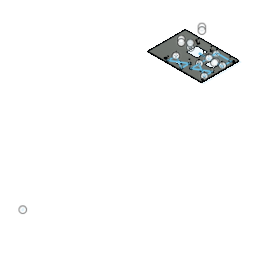
lid (Autodesk Fusion 360 design; units mm, degrees)
Autodesk Fusion 360 part; units mm, degrees
note: some values were not read from the file. Chosen so that the rebuilt part matches the saved one: which bodies a step acts on. Set by a fixed rule: which sketch regions a step uses; which face or edge a step refers to.
sketch "Sketch1" plane through (0, 0, 0) normal (0, 0, 1) x (1, 0, 0)
sketch "Sketch2" plane through (0, 0, 0) normal (1, 0, 0) x (0, 1, 0)
  line L0 (32, 8.9863) -> (32, 4)
  line L1 (-0.5157, 4) -> (-0.5157, 8.9863)
  circle A0 centre (-249.9, -99.15) radius 0.8
  constraint vertical L0
  constraint vertical L1
sketch "Sketch3" plane through (0, 0, 0) normal (0, 0, 1) x (1, 0, 0)
  circle A0 centre (4, 3.7) radius 0.8
extrude "Extrude1" add sketch "Sketch3" along normal blind 5 makes body 1
extrude "Extrude2" add 1 faces at (3.8681, 4.0199, 5) along direction (0, 0, 1) blind 1.5 on bodies 1 bodies 1
move_body "Move1" bodies 1 to x (1, 0, 0) y (0, 1, 0) z (0, 0, 1) at (0, 10, 0)
copy_body "CopyPasteBodies1" bodies 1 makes body 2
copy_body "CopyPasteBodies2" bodies 2 makes body 3
move_body "Move2" bodies 3 to x (1, 0, 0) y (0, 1, 0) z (0, 0, 1) at (0, -10, 0)
move_body "Move3" bodies 2 to x (1, 0, 0) y (0, 1, 0) z (0, 0, 1) at (0, 2.7, 0)
copy_body "CopyPasteBodies3" bodies 3 makes body 4
move_body "Move4" bodies 4 to x (1, 0, 0) y (0, 1, 0) z (0, 0, 1) at (21, 0, 0)
move_body "Move5" bodies 1 to x (1, 0, 0) y (0, 1, 0) z (0, 0, 1) at (21, 2.7, 0)
copy_body "CopyPasteBodies4" bodies 1 2 3 4 makes body 5 makes body 6 makes body 7 makes body 8
move_body "Move6" bodies 5 6 7 8 to x (1, 0, 0) y (0, 1, 0) z (0, 0, 1) at (26, 0, 0)
sketch "Sketch4" plane through (0, 0, 0) normal (0, 0, 1) x (1, 0, 0)
  line L0 (-9.0529, 25.1435) -> (80, 25.1435)
  line L1 (80, 25.1435) -> (80, -35)
  line L2 (80, -35) -> (-9.0529, -35)
  line L3 (-9.0529, -35) -> (-9.0529, 25.1435)
  constraint horizontal L0
  constraint vertical L1
  constraint horizontal L2
  constraint vertical L3
move_body "Move7" bodies 5 6 7 8 to x (1, 0, 0) y (0, 1, 0) z (0, 0, 1) at (1, 0, 0)
sketch "Sketch5" plane through (0, 0, 0) normal (0, 0, 1) x (1, 0, 0)
  line L0 (38.2, 17.2) -> (60.7999, 17.2)
  line L1 (60.7999, 17.2) -> (60.7999, 2.9046)
  line L2 (60.7999, 2.9046) -> (38.2, 2.9046)
  line L3 (38.2, 2.9046) -> (38.2, 17.2)
  line L4 (60.7999, 2.9046) -> (25.8, 2.9046)
  line L5 (25.8, 2.9046) -> (25.8, 2.9)
  line L6 (25.8, 2.9) -> (60.7999, 2.9)
  line L7 (60.7999, 2.9) -> (60.7999, 2.9046)
  constraint horizontal L0
  constraint vertical L1
  constraint horizontal L2
  constraint vertical L3
  constraint horizontal L4
  constraint vertical L5
  constraint horizontal L6
  constraint vertical L7
move_body "Move8" bodies 1 4 8 6 2 5 7 3 to x (1, 0, 0) y (0, 1, 0) z (0, 0, 1) at (10, 0, 0)
copy_body "CopyPasteBodies5" bodies 5 6 7 8 makes body 9 makes body 10 makes body 11 makes body 12
move_body "Move9" bodies 9 10 11 12 to x (1, 0, 0) y (0, 1, 0) z (0, 0, 1) at (0, -27, 0)
copy_body "CopyPasteBodies6" bodies 9 10 11 12 makes body 13 makes body 14 makes body 15 makes body 16
move_body "Move10" bodies 13 14 15 16 to x (1, 0, 0) y (0, 1, 0) z (0, 0, 1) at (-27, 0, 0)
move_body "Move11" bodies 3 15 1 4 14 2 13 16 to x (1, 0, 0) y (0, 1, 0) z (0, 0, 1) at (-2, 0, 0)
sketch "Sketch6" plane through (0, 0, 0) normal (0, 0, 1) x (1, 0, 0)
move_body "Move12" bodies 14 11 4 7 3 2 8 5 13 12 9 6 1 16 15 10 to x (1, 0, 0) y (0, 1, 0) z (0, 0, 1) at (-2, 0, 0)
extrude "Extrude3" add sketch "Sketch4" against normal blind 1 bodies 1 2 3 4 5 6 7 8 9 10 11 12 13 14 15 16
sketch "Sketch7" plane through (0, 0, 0) normal (0, 0, 1) x (-1, 0, 0)
  circle A0 centre (-10, 23.3) radius 0.8
  circle A1 centre (-31, 10.6) radius 0.8
  circle A2 centre (-39, 23.3) radius 0.8
  circle A3 centre (-60, 10.6) radius 0.8
  circle A4 centre (-39, -3.7) radius 0.8
  circle A5 centre (-60, -16.4) radius 0.8
  circle A6 centre (-10, -3.7) radius 0.8
  circle A7 centre (-31, -16.4) radius 0.8
  circle A8 centre (-10, -16.4) radius 0.8
  circle A9 centre (-31, -3.7) radius 0.8
  circle A10 centre (-39, -16.4) radius 0.8
  circle A11 centre (-60, -3.7) radius 0.8
  circle A12 centre (-39, 10.6) radius 0.8
  circle A13 centre (-60, 23.3) radius 0.8
  circle A14 centre (-10, 10.6) radius 0.8
  circle A15 centre (-31, 23.3) radius 0.8
  line L0 (9.0529, 35) -> (-80, 35)
  line L1 (-80, 35) -> (-80, -25.1435)
  line L2 (-80, -25.1435) -> (9.0529, -25.1435)
  line L3 (9.0529, -25.1435) -> (9.0529, 35)
  line L4 (-10, -16.4) -> (-28.4563, -16.4)
  line L5 (-28.4563, -16.4) -> (-28.4563, -3.2)
  line L6 (-28.4563, -3.2) -> (-10, -3.2)
  line L7 (-10, -3.2) -> (-10, -16.4)
  constraint horizontal L4
  constraint vertical L5
  constraint horizontal L6
  constraint vertical L7
  constraint coincident A8.centre L4.start
sketch "Sketch8" plane through (0, 0, 0) normal (0, 0, 1) x (1, 0, 0)
  line L0 (49.5, 4.5) -> (49.5, 2.2044)
  constraint vertical L0
sketch "Sketch9" plane through (0, 0, 0) normal (0, 0, 1) x (1, 0, 0)
  line L0 (12.5, -2) -> (28.5, -2)
  line L1 (28.5, -2) -> (28.5, 14)
  line L2 (28.5, 14) -> (12.5, 14)
  line L3 (12.5, 14) -> (12.5, -2)
  line L4 (28.5, 14) -> (12.5, 14)
  line L5 (12.5, 14) -> (12.5, -2)
  line L6 (12.5, -2) -> (28.5, -2)
  line L7 (28.5, -2) -> (28.5, 14)
  line L8 (12.5, -2) -> (28.5, -2)
  line L9 (28.5, -2) -> (28.5, 14)
  line L10 (28.5, 14) -> (12.5, 14)
  line L11 (12.5, 14) -> (12.5, -2)
  line L12 (12.5, 14) -> (28.5, 14)
  line L13 (28.5, 14) -> (28.5, -2)
  line L14 (28.5, -2) -> (12.5, -2)
  line L15 (12.5, -2) -> (12.5, 14)
  constraint horizontal L0
  constraint vertical L1
  constraint horizontal L2
  constraint vertical L3
  constraint horizontal L4
  constraint vertical L5
  constraint horizontal L6
  constraint vertical L7
  constraint horizontal L8
  constraint vertical L9
  constraint horizontal L10
  constraint vertical L11
  constraint horizontal L12
  constraint vertical L13
  constraint horizontal L14
  constraint vertical L15
extrude "Extrude4" cut sketch "Sketch9" along normal blind 1 and the other way blind 7 bodies 1
sketch "Sketch10" plane through (0, 0, 0) normal (0, 0, 1) x (-1, 0, 0)
  line L0 (-39, -15.6) -> (-39, -4.5)
  constraint vertical L0
sketch "Sketch11" plane through (0, 0, 0) normal (0, 0, 1) x (-1, 0, 0)
  line L0 (-39, -4.5) -> (-60, -4.5)
  constraint horizontal L0
sketch "Sketch12" plane through (0, 0, 0) normal (0, 0, 1) x (1, 0, 0)
  line L0 (43.75, 4.5) -> (55.25, 4.5)
  line L1 (55.25, 4.5) -> (55.25, -7)
  line L2 (55.25, -7) -> (43.75, -7)
  line L3 (43.75, -7) -> (43.75, 4.5)
  constraint horizontal L0
  constraint vertical L1
  constraint horizontal L2
  constraint vertical L3
extrude "Extrude5" cut sketch "Sketch12" along normal blind 2 and the other way blind 4 bodies 1
sketch "Sketch13" plane through (0, 0, 0) normal (0, 0, 1) x (1, 0, 0)
  line L0 (39, 2.9) -> (39, -11)
  constraint vertical L0
move_face "MoveFace1" to x (1, 0, 0) y (0, 1, 0) z (0, 0, 1) at (0, 0, 6) 1 faces at (30.3174, 15.9829, 4.3333) on bodies 1
split "Split1" by plane through (0, 0, 0) normal (0, 0, 1) bodies 1 makes body 17 at (9.201, -23.3399, 4.3333) makes body 18 at (10.796, -10.6797, 4.3333) makes body 19 at (31.796, -10.6797, 4.3333) makes body 20 at (60.365, -22.5881, 2.1667) makes body 21 at (39.365, -22.5881, 2.1667) makes body 22 at (39.1389, -9.8122, 2.1667) makes body 23 at (60.1389, -9.8122, 2.1667) makes body 24 at (60.1389, 4.4878, 2.1667) makes body 25 at (39.1389, 4.4878, 2.1667) makes body 26 at (39.0995, 15.6062, 2.1667) makes body 27 at (60.0995, 15.6062, 2.1667) makes body 28 at (31.796, 3.6203, 4.3333) makes body 29 at (10.796, 3.6203, 4.3333) makes body 30 at (9.201, 16.3601, 4.3333) makes body 31 at (30.3174, 15.9829, 4.3333) makes body 32 at (30.201, -23.3399, 4.3333)
move_face "MoveFace2" to x (1, 0, 0) y (0, 1, 0) z (0, 0, 1) at (0, -7, 0) 4 faces at (9.201, -23.3399, 4.3333) (10.796, -10.6797, 4.3333) (31.796, -10.6797, 4.3333) (30.201, -23.3399, 4.3333) on bodies 17 18 19 32
move_face "MoveFace3" to x (1, 0, 0) y (0, 1, 0) z (0, 0, 1) at (0, -1, 0) 8 faces at (39.1389, -9.8122, 2.1667) (60.1389, -9.8122, 2.1667) (60.365, -22.5881, 2.1667) (39.365, -22.5881, 2.1667) (30.201, -17.6399, 4.3333) (9.201, -17.6399, 4.3333) (9.201, -30.3399, 4.3333) (30.201, -30.3399, 4.3333) on bodies 17 18 19 20 21 22 23 32
sketch "Sketch14" plane through (0, 0, 0) normal (0, 0, 1) x (-1, 0, 0)
  line L0 (-10, 19.4) -> (-10, 31.3)
  line L1 (-10, 31.3) -> (-31, 18.6)
  line L2 (-31, 18.6) -> (-31, 31.3)
  line L3 (-31, 31.3) -> (-10, 18.6)
  constraint vertical L0
  constraint parallel L0 L2
hole "Hole1" at (20.5009, -24.9504, 0) direction (0, 0, -1) diameter 5.55 depth 5 tip angle 118 bodies 1
sketch "Sketch15" plane through (0, 0, 0) normal (0, 0, 1) x (-1, 0, 0)
  line L0 (-39, 11.6) -> (-39, 24.3)
  line L1 (-39, 24.3) -> (-60, 11.6)
  line L2 (-60, 11.6) -> (-60, 24.3)
  line L3 (-60, 24.3) -> (-39, 11.6)
  constraint vertical L0
  constraint parallel L0 L2
sketch "Sketch16" plane through (0, 0, 0) normal (0, 0, 1) x (-1, 0, 0)
  line L0 (-50.4991, 15.8331) -> (-48.5009, 15.8331)
  line L1 (-48.5009, 15.8331) -> (-48.5009, 20.0669)
  line L2 (-48.5009, 20.0669) -> (-50.4991, 20.0669)
  line L3 (-50.4991, 20.0669) -> (-50.4991, 15.8331)
  line L4 (-50.4991, 15.8331) -> (-48.5009, 20.0669) construction
  line L5 (-48.5009, 15.8331) -> (-50.4991, 20.0669) construction
  point P0 (-49.5, 17.95)
  constraint horizontal L0
  constraint perpendicular L0 L1
  constraint parallel L0 L2
  constraint parallel L1 L3
  constraint coincident L4 P0
  constraint coincident L5 P0
extrude "Extrude6" cut sketch "Sketch16" along normal blind 1.5 and the other way blind 1.5 bodies 1
sketch "Sketch17" plane through (0, 0, 0) normal (1, 0, 0) x (0, 1, 0)
  line L0 (3.7, 0, 10) -> (3.7, 6.5, 10)
chamfer "Chamfer2" distance 0.25 angle 45 16 edges at (38.2541, -11.8893, 6.5) (9.2541, -18.8893, 6.5) (59.2541, 3.4107, 6.5) (9.2541, -31.5893, 6.5) (59.2541, -11.8893, 6.5) (30.2541, -18.8893, 6.5) (30.2541, 16.1107, 6.5) (30.2541, -31.5893, 6.5) (38.2541, 3.4107, 6.5) (38.2541, 16.1107, 6.5) (9.2541, 3.4107, 6.5) (9.2541, 16.1107, 6.5) (59.2541, -24.5893, 6.5) (59.2541, 16.1107, 6.5) (30.2541, 3.4107, 6.5) (38.2541, -24.5893, 6.5) on bodies 2 3 4 5 6 7 8 17 18 19 20 21 22 23 24 25 26 27 28 29 30 31 32
fillet "Fillet1" radius 0.1 4 edges at (43.75, -7, -0.5) (43.75, 4.5, -0.5) (55.25, -7, -0.5) (55.25, 4.5, -0.5) on bodies 1
fillet "Fillet2" radius 0.1 4 edges at (48.5009, -15.8331, -0.5) (50.4991, -15.8331, -0.5) (48.5009, -20.0669, -0.5) (50.4991, -20.0669, -0.5) on bodies 1
fillet "Fillet3" radius 0.1 4 edges at (28.5, -2, -0.5) (28.5, 14, -0.5) (12.5, 14, -0.5) (12.5, -2, -0.5) on bodies 1
fillet "Fillet6" radius 0.075 1 edges at (17.9137, -23.9469, 0) on bodies 1
sketch "Sketch18" plane through (0, 0, 0) normal (0, 0, 1) x (-1, 0, 0)
  circle A0 centre (-60, 24.3) radius 1.2728
sketch "Sketch19" plane through (0, 0, 0) normal (0, 0, 1) x (1, 0, 0)
  circle A0 centre (10, 16.4) radius 1.8028
extrude "Extrude7" add sketch "Sketch19" along normal blind 1.5 separate body makes body 33
sketch "Sketch20" plane through (0, 0, 0) normal (0, 0, 1) x (-1, 0, 0)
  circle A0 centre (-31, -16.4) radius 1.75
  dimension "d38" = 3.5
  measures "d38" diameter of A0
extrude "Extrude8" add sketch "Sketch20" along normal blind 1.5 separate body makes body 34
sketch "Sketch21" plane through (0, 0, 0) normal (0, 0, 1) x (-1, 0, 0)
  circle A0 centre (-39, -16.4) radius 1.75
  dimension "d41" = 3.5
  measures "d41" diameter of A0
extrude "Extrude9" add sketch "Sketch21" along normal blind 1.5 separate body makes body 35
sketch "Sketch22" plane through (0, 0, 0) normal (0, 0, 1) x (-1, 0, 0)
  circle A0 centre (-39, -3.7) radius 1.75
  dimension "d44" = 3.5
  measures "d44" diameter of A0
extrude "Extrude10" add sketch "Sketch22" along normal blind 1.5 separate body makes body 36
sketch "Sketch23" plane through (0, 0, 0) normal (0, 0, 1) x (-1, 0, 0)
  circle A0 centre (-31, -3.7) radius 1.75
  dimension "d47" = 3.5
  measures "d47" diameter of A0
extrude "Extrude11" add sketch "Sketch23" along normal blind 1.5 separate body makes body 37
sketch "Sketch24" plane through (0, 0, 0) normal (0, 0, 1) x (-1, 0, 0)
  circle A0 centre (-39, 11.6) radius 1.75
  dimension "d50" = 3.5
  measures "d50" diameter of A0
extrude "Extrude12" add sketch "Sketch24" along normal blind 1.5 separate body makes body 38
sketch "Sketch25" plane through (0, 0, 0) normal (0, 0, 1) x (-1, 0, 0)
  circle A0 centre (-60, -16.4) radius 1.75
  dimension "d53" = 3.5
  measures "d53" diameter of A0
extrude "Extrude13" add sketch "Sketch25" along normal blind 1.5 separate body makes body 39
sketch "Sketch26" plane through (0, 0, 0) normal (0, 0, 1) x (-1, 0, 0)
  circle A0 centre (-60, -3.7) radius 1.75
  dimension "d56" = 3.5
  measures "d56" diameter of A0
extrude "Extrude14" add sketch "Sketch26" along normal blind 1.5 separate body makes body 40
sketch "Sketch27" plane through (0, 0, 0) normal (0, 0, 1) x (-1, 0, 0)
  circle A0 centre (-60, 11.6) radius 1.75
  dimension "d59" = 3.5
  measures "d59" diameter of A0
extrude "Extrude15" add sketch "Sketch27" along normal blind 1.5 separate body makes body 41
sketch "Sketch28" plane through (0, 0, 0) normal (0, 0, 1) x (-1, 0, 0)
  circle A0 centre (-60, 24.3) radius 1.75
  dimension "d62" = 3.5
  measures "d62" diameter of A0
extrude "Extrude16" add sketch "Sketch28" along normal blind 1.5 separate body makes body 42
sketch "Sketch29" plane through (0, 0, 0) normal (0, 0, 1) x (-1, 0, 0)
  circle A0 centre (-39, 24.3) radius 1.75
  dimension "d65" = 3.5
  measures "d65" diameter of A0
extrude "Extrude17" add sketch "Sketch29" along normal blind 1.5 separate body makes body 43
sketch "Sketch30" plane through (0, 0, 0) normal (0, 0, 1) x (-1, 0, 0)
  circle A0 centre (-31, 18.6) radius 1.7499
extrude "Extrude18" cut sketch "Sketch30" along normal blind 1.5 bodies 19
sketch "Sketch31" plane through (0, 0, 0) normal (0, 0, 1) x (-1, 0, 0)
  circle A0 centre (-10, -3.7) radius 1.75
  dimension "d70" = 3.5
  measures "d70" diameter of A0
extrude "Extrude19" add sketch "Sketch31" along normal blind 1.5 separate body makes body 44
sketch "Sketch32" plane through (0, 0, 0) normal (0, 0, 1) x (-1, 0, 0)
  circle A0 centre (-10, 18.6) radius 1.75
  dimension "d73" = 3.5
  measures "d73" diameter of A0
extrude "Extrude20" add sketch "Sketch32" along normal blind 1.5 separate body makes body 45
sketch "Sketch33" plane through (0, 0, 0) normal (0, 0, 1) x (-1, 0, 0)
  circle A0 centre (-31, 18.6) radius 1.75
  dimension "d76" = 3.5
  measures "d76" diameter of A0
extrude "Extrude21" add sketch "Sketch33" along normal blind 1.5 bodies 1 19
sketch "Sketch34" plane through (0, 0, 0) normal (0, 0, 1) x (-1, 0, 0)
  circle A0 centre (-31, 31.3) radius 1.75
  dimension "d79" = 3.5
  measures "d79" diameter of A0
extrude "Extrude22" add sketch "Sketch34" along normal blind 1.5 separate body makes body 46
sketch "Sketch35" plane through (0, 0, 0) normal (0, 0, 1) x (-1, 0, 0)
  circle A0 centre (-10, 31.3) radius 1.75
  dimension "d82" = 3.5
  measures "d82" diameter of A0
extrude "Extrude23" add sketch "Sketch35" along normal blind 1.5 separate body makes body 47
fillet "Fillet7" radius 0.5 4 edges at (-9.0529, 25.1435, -0.5) (80, 25.1435, -0.5) (80, -35, -0.5) (-9.0529, -35, -0.5) on bodies 1
sketch "Sketch36" plane through (0, 0, 0) normal (0, 0, 1) x (-1, 0, 0)
  line L0 (-1.7, 34.5) -> (-79.5, 34.5)
  line L1 (-79.5, 34.5) -> (-79.5, -24.7)
  line L2 (-79.5, -24.7) -> (-1.7, -24.7)
  line L3 (-1.7, -24.7) -> (-1.7, 34.5)
  constraint horizontal L0
  constraint vertical L1
  constraint horizontal L2
  constraint vertical L3
extrude "Extrude24" cut sketch "Sketch36" against normal blind 0.5 bodies 1 makes body 48 at (31.796, -18.5203, 3.0833)
move_body "Move13" bodies 45 18 47 17 44 29 30 33 34 31 26 35 39 27 24 40 25 36 28 37 48 38 22 43 21 23 41 20 42 32 46 to x (1, 0, 0) y (0, 1, 0) z (0, 0, 1) at (0, 0, -0.5)
move_face "MoveFace4" by (10.2, 0, 0) 1 faces at (-9.0529, -14.7855, -0.3333) on bodies 1
move_face "MoveFace5" by (10.2, 0, 0) 1 faces at (80, 4.929, -0.3333) on bodies 1
move_face "MoveFace6" by (10.2, 0, 0) 1 faces at (79.5, 4.9667, -0.3333) on bodies 1
move_face "MoveFace7" by (-20.4, 0, 0) 2 faces at (89.7, 4.9667, -0.3333) (90.2, 4.929, -0.3333) on bodies 1
move_face "MoveFace8" by (-20.4, 0, 0) 2 faces at (1.7, -14.7667, -0.3333) (1.1471, -14.7855, -0.3333) on bodies 1
sketch "Sketch37" plane through (0, 0, -0.5) normal (0, 0, 1) x (-1, 0, 0)
  circle A0 centre (-20.5009, 24.9504) radius 2.775
  arc A1 (-12.6, -14) -> (-12.5, -13.9) centre (-12.6, -13.9) ccw
  line L0 (-12.6, -14) -> (-28.4, -14)
  arc A2 (-28.5, -13.9) -> (-28.4, -14) centre (-28.4, -13.9) ccw
  line L1 (-28.5, -13.9) -> (-28.5, 1.9)
  arc A3 (-28.4, 2) -> (-28.5, 1.9) centre (-28.4, 1.9) ccw
  line L2 (-28.4, 2) -> (-12.6, 2)
  arc A4 (-12.5, 1.9) -> (-12.6, 2) centre (-12.6, 1.9) ccw
  line L3 (-12.5, 1.9) -> (-12.5, -13.9)
  arc A5 (-48.5009, 19.9669) -> (-48.6009, 20.0669) centre (-48.6009, 19.9669) ccw
  line L4 (-48.5009, 19.9669) -> (-48.5009, 15.9331)
  arc A6 (-48.6009, 15.8331) -> (-48.5009, 15.9331) centre (-48.6009, 15.9331) ccw
  line L5 (-48.6009, 15.8331) -> (-50.3991, 15.8331)
  arc A7 (-50.4991, 15.9331) -> (-50.3991, 15.8331) centre (-50.3991, 15.9331) ccw
  line L6 (-50.4991, 15.9331) -> (-50.4991, 19.9669)
  arc A8 (-50.3991, 20.0669) -> (-50.4991, 19.9669) centre (-50.3991, 19.9669) ccw
  line L7 (-50.3991, 20.0669) -> (-48.6009, 20.0669)
  arc A9 (-43.85, -4.5) -> (-43.75, -4.4) centre (-43.85, -4.4) ccw
  line L8 (-43.85, -4.5) -> (-55.15, -4.5)
  arc A10 (-55.25, -4.4) -> (-55.15, -4.5) centre (-55.15, -4.4) ccw
  line L9 (-55.25, -4.4) -> (-55.25, 6.9)
  arc A11 (-55.15, 7) -> (-55.25, 6.9) centre (-55.15, 6.9) ccw
  line L10 (-55.15, 7) -> (-43.85, 7)
  arc A12 (-43.75, 6.9) -> (-43.85, 7) centre (-43.85, 6.9) ccw
  line L11 (-43.75, 6.9) -> (-43.75, -4.4)
  line L12 (18.7, -24.7) -> (18.7, 34.5)
  line L13 (18.7, 34.5) -> (-69.3, 34.5)
  line L14 (-69.3, 34.5) -> (-69.3, -24.7)
  line L15 (-69.3, -24.7) -> (18.7, -24.7)
  line L16 (-8.2, -18.2) -> (-32.7552, -18.2)
  line L17 (-32.7552, -18.2) -> (-32.7552, -1.944)
  line L18 (-32.7552, -1.944) -> (-8.2, -1.944)
  line L19 (-8.2, -1.944) -> (-8.2, -18.2)
  line L20 (-10, -16.4) -> (-31, -16.4)
  line L21 (-10, -3.7) -> (-31, -3.7)
  constraint horizontal L16
  constraint vertical L17
  constraint horizontal L18
  constraint vertical L19
  constraint parallel L0 L20
  constraint perpendicular L1 L21
move_face "OffsetFaces1" offset 2.3 1 faces at (17.8667, 14, -0.6667) on bodies 1
move_face "OffsetFaces2" offset -2.3 1 faces at (17.8667, -2, -0.8333) on bodies 1
sketch "Sketch38" plane through (0, 0, -0.5) normal (0, 0, 1) x (-1, 0, 0)
  line L0 (-12.5, 4.2) -> (-12.5, -11.6)
  arc A0 (-12.6, -11.7) -> (-12.5, -11.6) centre (-12.6, -11.6) ccw
  line L1 (-12.6, -11.7) -> (-28.4, -11.7)
  arc A1 (-28.5, -11.6) -> (-28.4, -11.7) centre (-28.4, -11.6) ccw
  line L2 (-28.5, -11.6) -> (-28.5, 4.2)
  arc A2 (-28.4, 4.3) -> (-28.5, 4.2) centre (-28.4, 4.2) ccw
  line L3 (-28.4, 4.3) -> (-12.6, 4.3)
  arc A3 (-12.5, 4.2) -> (-12.6, 4.3) centre (-12.6, 4.2) ccw
  circle A4 centre (-20.5009, 24.9504) radius 2.775
  arc A5 (-48.5009, 19.9669) -> (-48.6009, 20.0669) centre (-48.6009, 19.9669) ccw
  line L4 (-48.5009, 19.9669) -> (-48.5009, 15.9331)
  arc A6 (-48.6009, 15.8331) -> (-48.5009, 15.9331) centre (-48.6009, 15.9331) ccw
  line L5 (-48.6009, 15.8331) -> (-50.3991, 15.8331)
  arc A7 (-50.4991, 15.9331) -> (-50.3991, 15.8331) centre (-50.3991, 15.9331) ccw
  line L6 (-50.4991, 15.9331) -> (-50.4991, 19.9669)
  arc A8 (-50.3991, 20.0669) -> (-50.4991, 19.9669) centre (-50.3991, 19.9669) ccw
  line L7 (-50.3991, 20.0669) -> (-48.6009, 20.0669)
  arc A9 (-43.85, -4.5) -> (-43.75, -4.4) centre (-43.85, -4.4) ccw
  line L8 (-43.85, -4.5) -> (-55.15, -4.5)
  arc A10 (-55.25, -4.4) -> (-55.15, -4.5) centre (-55.15, -4.4) ccw
  line L9 (-55.25, -4.4) -> (-55.25, 6.9)
  arc A11 (-55.15, 7) -> (-55.25, 6.9) centre (-55.15, 6.9) ccw
  line L10 (-55.15, 7) -> (-43.85, 7)
  arc A12 (-43.75, 6.9) -> (-43.85, 7) centre (-43.85, 6.9) ccw
  line L11 (-43.75, 6.9) -> (-43.75, -4.4)
  line L12 (18.7, -24.7) -> (18.7, 34.5)
  line L13 (18.7, 34.5) -> (-69.3, 34.5)
  line L14 (-69.3, 34.5) -> (-69.3, -24.7)
  line L15 (-69.3, -24.7) -> (18.7, -24.7)
  line L16 (18.7, -24.7) -> (15.2004, -24.7)
  line L17 (15.2004, -24.7) -> (15.2004, 34.5)
  line L18 (15.2004, 34.5) -> (18.7, 34.5)
  line L19 (18.7, 34.5) -> (18.7, -24.7)
  line L20 (18.7, 34.5) -> (-65.7727, 34.5)
  line L21 (-65.7727, 34.5) -> (-65.7727, 31)
  line L22 (-65.7727, 31) -> (18.7, 31)
  line L23 (18.7, 31) -> (18.7, 34.5)
  line L24 (18.7, -24.7) -> (-69.2998, -24.7)
  line L25 (-69.2998, -24.7) -> (-69.2998, -21.2)
  line L26 (-69.2998, -21.2) -> (18.7, -21.2)
  line L27 (18.7, -21.2) -> (18.7, -24.7)
  line L28 (-69.3, -24.7) -> (-65.8, -24.7)
  line L29 (-65.8, -24.7) -> (-65.8, -21.2)
  line L30 (-65.8, -21.2) -> (-69.3, -21.2)
  line L31 (-69.3, -21.2) -> (-69.3, -24.7)
  line L32 (-69.3, 34.5) -> (-65.8, 34.5)
  line L33 (-65.8, 34.5) -> (-65.8, 31)
  line L34 (-65.8, 31) -> (-69.3, 31)
  line L35 (-69.3, 31) -> (-69.3, 34.5)
  circle A13 centre (-65.7727, 31) radius 1.55
  dimension "d91" = 3.5
  dimension "d92" = 3.5
  dimension "d93" = 3.5
  dimension "d94" = 3.1
  constraint horizontal L16
  constraint vertical L17
  constraint horizontal L18
  constraint vertical L19
  constraint coincident L13 L17.end
  constraint coincident L12.start L15.end
  constraint horizontal L20
  constraint vertical L21
  constraint horizontal L22
  constraint vertical L23
  constraint coincident L12.end L13.start
  constraint horizontal L24
  constraint vertical L25
  constraint horizontal L26
  constraint vertical L27
  constraint horizontal L28
  constraint vertical L29
  constraint horizontal L30
  constraint vertical L31
  constraint coincident L14.end L15.start
  constraint horizontal L32
  constraint vertical L33
  constraint horizontal L34
  constraint vertical L35
  constraint coincident L13.end L14.start
  constraint coincident L21.end L22.start
  measures "d91" distance of L12.end L22.end
  measures "d92" distance of L12.start L26.end
  measures "d93" distance of L14.end L28.end
  measures "d94" diameter of A13
sketch "Sketch39" plane through (0, 0, -0.5) normal (0, 0, 1) x (-1, 0, 0)
  line L0 (-12.5, 4.2) -> (-12.5, -11.6)
  arc A0 (-12.6, -11.7) -> (-12.5, -11.6) centre (-12.6, -11.6) ccw
  line L1 (-12.6, -11.7) -> (-28.4, -11.7)
  arc A1 (-28.5, -11.6) -> (-28.4, -11.7) centre (-28.4, -11.6) ccw
  line L2 (-28.5, -11.6) -> (-28.5, 4.2)
  arc A2 (-28.4, 4.3) -> (-28.5, 4.2) centre (-28.4, 4.2) ccw
  line L3 (-28.4, 4.3) -> (-12.6, 4.3)
  arc A3 (-12.5, 4.2) -> (-12.6, 4.3) centre (-12.6, 4.2) ccw
  circle A4 centre (-20.5009, 24.9504) radius 2.775
  arc A5 (-48.5009, 19.9669) -> (-48.6009, 20.0669) centre (-48.6009, 19.9669) ccw
  line L4 (-48.5009, 19.9669) -> (-48.5009, 15.9331)
  arc A6 (-48.6009, 15.8331) -> (-48.5009, 15.9331) centre (-48.6009, 15.9331) ccw
  line L5 (-48.6009, 15.8331) -> (-50.3991, 15.8331)
  arc A7 (-50.4991, 15.9331) -> (-50.3991, 15.8331) centre (-50.3991, 15.9331) ccw
  line L6 (-50.4991, 15.9331) -> (-50.4991, 19.9669)
  arc A8 (-50.3991, 20.0669) -> (-50.4991, 19.9669) centre (-50.3991, 19.9669) ccw
  line L7 (-50.3991, 20.0669) -> (-48.6009, 20.0669)
  arc A9 (-43.85, -4.5) -> (-43.75, -4.4) centre (-43.85, -4.4) ccw
  line L8 (-43.85, -4.5) -> (-55.15, -4.5)
  arc A10 (-55.25, -4.4) -> (-55.15, -4.5) centre (-55.15, -4.4) ccw
  line L9 (-55.25, -4.4) -> (-55.25, 6.9)
  arc A11 (-55.15, 7) -> (-55.25, 6.9) centre (-55.15, 6.9) ccw
  line L10 (-55.15, 7) -> (-43.85, 7)
  arc A12 (-43.75, 6.9) -> (-43.85, 7) centre (-43.85, 6.9) ccw
  line L11 (-43.75, 6.9) -> (-43.75, -4.4)
  line L12 (18.7, -24.7) -> (18.7, 34.5)
  line L13 (18.7, 34.5) -> (-69.3, 34.5)
  line L14 (-69.3, 34.5) -> (-69.3, -24.7)
  line L15 (-69.3, -24.7) -> (18.7, -24.7)
  line L16 (-69.3, -24.7) -> (-65.8, -24.7)
  line L17 (-65.8, -24.7) -> (-65.8, -21.2)
  line L18 (-65.8, -21.2) -> (-69.3, -21.2)
  line L19 (-69.3, -21.2) -> (-69.3, -24.7)
  circle A13 centre (-65.8, -21.2) radius 1.55
  dimension "d97" = 3.1
  constraint horizontal L16
  constraint vertical L17
  constraint horizontal L18
  constraint vertical L19
  constraint coincident L14.end L15.start
  constraint coincident L17.end L18.start
  measures "d97" diameter of A13
sketch "Sketch40" plane through (0, 0, -0.5) normal (0, 0, 1) x (-1, 0, 0)
  line L0 (-12.5, 4.2) -> (-12.5, -11.6)
  arc A0 (-12.6, -11.7) -> (-12.5, -11.6) centre (-12.6, -11.6) ccw
  line L1 (-12.6, -11.7) -> (-28.4, -11.7)
  arc A1 (-28.5, -11.6) -> (-28.4, -11.7) centre (-28.4, -11.6) ccw
  line L2 (-28.5, -11.6) -> (-28.5, 4.2)
  arc A2 (-28.4, 4.3) -> (-28.5, 4.2) centre (-28.4, 4.2) ccw
  line L3 (-28.4, 4.3) -> (-12.6, 4.3)
  arc A3 (-12.5, 4.2) -> (-12.6, 4.3) centre (-12.6, 4.2) ccw
  circle A4 centre (-20.5009, 24.9504) radius 2.775
  arc A5 (-48.5009, 19.9669) -> (-48.6009, 20.0669) centre (-48.6009, 19.9669) ccw
  line L4 (-48.5009, 19.9669) -> (-48.5009, 15.9331)
  arc A6 (-48.6009, 15.8331) -> (-48.5009, 15.9331) centre (-48.6009, 15.9331) ccw
  line L5 (-48.6009, 15.8331) -> (-50.3991, 15.8331)
  arc A7 (-50.4991, 15.9331) -> (-50.3991, 15.8331) centre (-50.3991, 15.9331) ccw
  line L6 (-50.4991, 15.9331) -> (-50.4991, 19.9669)
  arc A8 (-50.3991, 20.0669) -> (-50.4991, 19.9669) centre (-50.3991, 19.9669) ccw
  line L7 (-50.3991, 20.0669) -> (-48.6009, 20.0669)
  arc A9 (-43.85, -4.5) -> (-43.75, -4.4) centre (-43.85, -4.4) ccw
  line L8 (-43.85, -4.5) -> (-55.15, -4.5)
  arc A10 (-55.25, -4.4) -> (-55.15, -4.5) centre (-55.15, -4.4) ccw
  line L9 (-55.25, -4.4) -> (-55.25, 6.9)
  arc A11 (-55.15, 7) -> (-55.25, 6.9) centre (-55.15, 6.9) ccw
  line L10 (-55.15, 7) -> (-43.85, 7)
  arc A12 (-43.75, 6.9) -> (-43.85, 7) centre (-43.85, 6.9) ccw
  line L11 (-43.75, 6.9) -> (-43.75, -4.4)
  line L12 (18.7, -24.7) -> (18.7, 34.5)
  line L13 (18.7, 34.5) -> (-69.3, 34.5)
  line L14 (-69.3, 34.5) -> (-69.3, -24.7)
  line L15 (-69.3, -24.7) -> (18.7, -24.7)
move_face "MoveFace9" by (-2, 0, 0) 2 faces at (69.3, -14.7667, -0.1667) (69.8, 4.929, -0.3333) on bodies 1
move_face "MoveFace10" by (-1.5, 0, 0) 2 faces at (67.3, -14.7667, -0.1667) (67.8, 4.929, -0.3333) on bodies 1
move_face "MoveFace11" by (0, 0, -3.5) 2 faces at (-18.7, 4.9667, -0.1667) (-19.2529, 4.929, -0.6667) on bodies 1
sketch "Sketch41" plane through (0, 0, -0.5) normal (0, 0, 1) x (-1, 0, 0)
  line L0 (-65.8, -24.7) -> (-62.3, -24.7)
  line L1 (-62.3, -24.7) -> (-62.3, -19.6)
  line L2 (-62.3, -19.6) -> (-65.8, -19.6)
  line L3 (-65.8, -19.6) -> (-65.8, -24.7)
  circle A0 centre (-62.3, -19.6) radius 1.55
  line L4 (-61.1, -17.8) -> (-60.4, -18.3)
  circle A1 centre (-62.3, -19.6) radius 2.9
  dimension "d102" = 3.1
  dimension "d103" = 5.8
  constraint horizontal L0
  constraint vertical L1
  constraint horizontal L2
  constraint vertical L3
  constraint coincident L1.end L2.start
  constraint concentric A0 A1
  measures "d102" diameter of A0
  measures "d103" diameter of A1
extrude "Extrude27" cut sketch "Sketch41" along normal blind 1.5 contours L1 L2 A0 A1 picked at (-63.3253, -17.382) bodies 39
sketch "Sketch42" plane through (0, 0, -0.5) normal (0, 0, 1) x (-1, 0, 0)
  line L0 (-65.8, -24.7) -> (-62.3, -24.7)
  line L1 (-62.3, -24.7) -> (-62.3, -19.6)
  line L2 (-62.3, -19.6) -> (-65.8, -19.6)
  line L3 (-65.8, -19.6) -> (-65.8, -24.7)
  circle A0 centre (-62.3, -19.6) radius 1.55
  dimension "d106" = 3.1
  constraint horizontal L0
  constraint vertical L1
  constraint horizontal L2
  constraint vertical L3
  constraint coincident L1.end L2.start
  measures "d106" diameter of A0
extrude "Extrude28" cut sketch "Sketch42" against normal blind 0.7 contours L1 L2 A0 | L1 L2 A0 bodies 1
sketch "Sketch43" plane through (0, 0, -0.5) normal (0, 0, 1) x (-1, 0, 0)
  line L0 (-65.8, 34.5) -> (-62.3, 34.5)
  line L1 (-62.3, 34.5) -> (-62.3, 29.4)
  line L2 (-62.3, 29.4) -> (-65.8, 29.4)
  line L3 (-65.8, 29.4) -> (-65.8, 34.5)
  circle A0 centre (-62.3, 29.4) radius 1.55
  dimension "d109" = 5.1
  dimension "d110" = 3.1
  constraint horizontal L0
  constraint vertical L1
  constraint horizontal L2
  constraint vertical L3
  constraint coincident L1.end L2.start
  measures "d109" distance of L0.start L2.end
  measures "d110" diameter of A0
extrude "Extrude29" cut sketch "Sketch43" against normal blind 0.6 contours L1 L2 A0 | L1 L2 A0 bodies 1
sketch "Sketch44" plane through (0, 0, -0.5) normal (0, 0, 1) x (-1, 0, 0)
  line L0 (-65.8, 34.5) -> (-4.3, 34.5)
  line L1 (-4.3, 34.5) -> (-4.3, 29.4)
  line L2 (-4.3, 29.4) -> (-65.8, 29.4)
  line L3 (-65.8, 29.4) -> (-65.8, 34.5)
  circle A0 centre (-4.3, 29.4) radius 1.55
  dimension "d113" = 61.5
  dimension "d114" = 5.1
  dimension "d115" = 3.1
  constraint horizontal L0
  constraint vertical L1
  constraint horizontal L2
  constraint vertical L3
  constraint coincident L1.end L2.start
  measures "d113" distance of L0.start L0.end
  measures "d114" distance of L0.start L2.end
  measures "d115" diameter of A0
extrude "Extrude30" cut sketch "Sketch44" against normal blind 0.6 contours L1 L2 A0 | L1 L2 A0 bodies 1
sketch "Sketch45" plane through (0, 0, -0.5) normal (0, 0, 1) x (-1, 0, 0)
  line L0 (-65.8, -24.7) -> (-4.3, -24.7)
  line L1 (-4.3, -24.7) -> (-4.3, -19.6)
  line L2 (-4.3, -19.6) -> (-65.8, -19.6)
  line L3 (-65.8, -19.6) -> (-65.8, -24.7)
  circle A0 centre (-4.3, -19.6) radius 1.55
  dimension "d118" = 61.5
  dimension "d119" = 5.1
  dimension "d120" = 3.1
  constraint horizontal L0
  constraint vertical L1
  constraint horizontal L2
  constraint vertical L3
  constraint coincident L1.end L2.start
  measures "d118" distance of L0.start L0.end
  measures "d119" distance of L0.start L2.end
  measures "d120" diameter of A0
extrude "Extrude31" cut sketch "Sketch45" against normal blind 0.6 contours L1 L2 A0 | L1 L2 A0 bodies 1
named bodies: "Top Right", "Top Left", "Bottom Left", "Bottom Right", "Top Right (1)", "Top Left (1)", "Bottom Left (1)", "Bottom Right (1)", "Top Right (1) (1)", "Top Left (1) (1)", "Bottom Left (1) (1)", "Bottom Right (1) (1)", "Top Right (1) (1) (1)", "Top Left (1) (1) (1)", "Bottom Left (1) (1) (1)", "Bottom Right (1) (1) (1)", "Top Right (2)", "Top Right (3)", "Top Right (4)", "Top Right (5)", "Top Right (6)", "Top Right (7)", "Top Right (8)", "Top Right (9)", "Top Right (10)", "Top Right (11)", "Top Right (12)", "Top Right (13)", "Top Right (14)", "Top Right (15)", "Top Right (16)"
